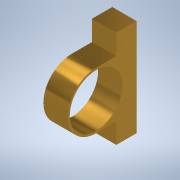
# Autodesk Inventor part: Abrazaderas tubo transparente
Saved by Autodesk Inventor 2020 (Build 240168000, 168)
## iProperties
Created: 2020-02-20
Part Number: Abrazaderas tubo transparente
Material: Latón, amarillo claro
Document SubType Name: Modeling
Designer: PabloGod
Density: 8.47 g/cm^3
Appearance: Latón - Satinado
Mass: 852.739 g
Surface Area: 242.366 cm^2
Volume: 100.678 cm^3
Author: PabloGod
Autodesk Inventor part; units mm, degrees
ref_plane "YZ Plane" through (0, 0, 0) normal (1, 0, 0) x (0, 1, 0)
ref_plane "XZ Plane" through (0, 0, 0) normal (0, 1, 0) x (-1, 0, 0)
ref_plane "XY Plane" through (0, 0, 0) normal (0, 0, 1) x (1, 0, 0)
sketch "Boceto1" plane through (0, 0, 0) normal (1, 0, 0) x (0, 1, 0)
  circle A0 centre (0, 0) radius 32.5
  arc A1 (35, 0) -> (-35, 0) centre (0, 0) ccw
  line L0 (-35, -25) -> (-60, -25)
  line L1 (-60, -50) -> (60, -50)
  line L2 (60, -50) -> (60, -25)
  line L3 (60, -25) -> (35, -25)
  line L4 (-35, 0) -> (-35, -25)
  line L5 (35, 0) -> (35, -25)
  line L6 (-60, -25) -> (-60, -50)
  dimension "d0" = 65
  dimension "d1" = 70
  dimension "d2" = 25
  dimension "d3" = 25
  dimension "d4" = 25
  dimension "d5" = 120
  dimension "d6" = 25
  dimension "d7" = 25
  constraints: 14 end point, 2 centre point, 2 point on circle, 2 point on line, 2 vertical, 1 coincident, 1 parallel
  measures "d0" diameter of A0
  measures "d1" diameter of A1
  measures "d2" distance of L4.start L0.start
  measures "d3" distance of L0.start L0.end
  measures "d4" distance of L0.end L1.start
  measures "d5" distance of L1.start L2.start
  measures "d6" distance of L2.start L3.start
  measures "d7" distance of L3.start L3.end
extrude "Extrusión1" add sketch "Boceto1" along normal mid plane 30
